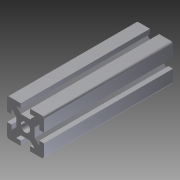
# Autodesk Inventor part: 5 in shooter standoff
Saved by Autodesk Inventor 2011 SP1 (Build 150282100, 282)
## iProperties
Created: 2012-01-20
Part Number: 5 in shooter standoff
Document SubType Name: Modeling
Designer: Christopher
Density: 1 g/cm^3
Author: Christopher
Autodesk Inventor part; units mm, degrees
ref_plane "YZ Plane" through (0, 0, 0) normal (1, 0, 0) x (0, 1, 0)
ref_plane "XZ Plane" through (0, 0, 0) normal (0, 1, 0) x (-1, 0, 0)
ref_plane "XY Plane" through (0, 0, 0) normal (0, 0, 1) x (1, 0, 0)
sketch "Sketch1" plane through (0, 0, 0) normal (0, 0, 1) x (1, 0, 0)
  line L0 (0, 15.875) -> (3.175, 15.875)
  line L1 (3.175, 15.875) -> (3.175, 19.05)
  line L2 (3.175, 19.05) -> (6.35, 15.875)
  line L3 (6.35, 15.875) -> (6.35, 9.525)
  line L4 (6.35, 9.525) -> (3.175, 6.35)
  line L5 (3.175, 6.35) -> (3.175, 9.525)
  line L6 (3.175, 9.525) -> (0, 9.525)
  line L7 (9.525, 0) -> (9.525, 3.175)
  line L8 (9.525, 3.175) -> (6.35, 3.175)
  line L9 (6.35, 3.175) -> (9.525, 6.35)
  line L10 (9.525, 6.35) -> (15.875, 6.35)
  line L11 (15.875, 6.35) -> (19.05, 3.175)
  line L12 (19.05, 3.175) -> (15.875, 3.175)
  line L13 (15.875, 3.175) -> (15.875, 0)
  line L14 (25.4, 9.525) -> (22.225, 9.525)
  line L15 (22.225, 9.525) -> (22.225, 6.35)
  line L16 (22.225, 6.35) -> (19.05, 9.525)
  line L17 (19.05, 9.525) -> (19.05, 15.875)
  line L18 (19.05, 15.875) -> (22.225, 19.05)
  line L19 (22.225, 19.05) -> (22.225, 15.875)
  line L20 (22.225, 15.875) -> (25.4, 15.875)
  line L21 (15.875, 25.4) -> (15.875, 22.225)
  line L22 (15.875, 22.225) -> (19.05, 22.225)
  line L23 (19.05, 22.225) -> (15.875, 19.05)
  line L24 (15.875, 19.05) -> (9.525, 19.05)
  line L25 (9.525, 19.05) -> (6.35, 22.225)
  line L26 (6.35, 22.225) -> (9.525, 22.225)
  line L27 (9.525, 22.225) -> (9.525, 25.4)
  circle A0 centre (12.7, 12.7) radius 3.175
  line L28 (0, 23.8125) -> (0, 15.875)
  line L29 (0, 9.525) -> (0, 1.5875)
  line L30 (9.525, 0) -> (1.5875, 0)
  line L31 (15.875, 0) -> (23.8125, 0)
  line L32 (25.4, 1.5875) -> (25.4, 9.525)
  line L33 (25.4, 15.875) -> (25.4, 23.8125)
  line L34 (23.8125, 25.4) -> (15.875, 25.4)
  line L35 (9.525, 25.4) -> (1.5875, 25.4)
  arc A1 (0, 1.5875) -> (1.5875, 0) centre (1.5875, 1.5875) ccw
  arc A2 (1.5875, 25.4) -> (0, 23.8125) centre (1.5875, 23.8125) ccw
  arc A3 (25.4, 23.8125) -> (23.8125, 25.4) centre (23.8125, 23.8125) ccw
  arc A4 (23.8125, 0) -> (25.4, 1.5875) centre (23.8125, 1.5875) ccw
  point P0 (0, 0)
  point P1 (25.4, 0)
  point P2 (0, 25.4)
  dimension "d5" = 6.35
  dimension "d7" = 12.7
  dimension "d8" = 3.175
  dimension "d9" = 3.175
  dimension "d13" = 360
  dimension "d15" = 6.35
  dimension "d16" = 1.5875
  constraints: 72 end point, 8 point on circle, 8 tangent, 6 point on line, 5 centre point, 5 collinear, 5 perpendicular, 3 equal radius, 2 parallel, 1 coincident, 61 other
  measures "d5" distance between parallel lines of L0 L6
  measures "d7" distance of L4.end L1.end
  measures "d8" distance from line of L1.end L0
  measures "d9" distance between parallel lines of L1 L3
  measures "d15" diameter of A0
  measures "d16" radius of A1
extrude "Extrusion2" add sketch "Sketch1" against normal blind 88.9
body "Solid1"
